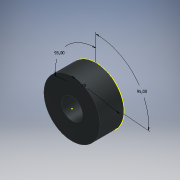
# Autodesk Inventor part: greggio tranciato
Saved by Autodesk Inventor 2018 (Build 220112000, 112)
## iProperties
Created: 2018-08-09
Part Number: greggio tranciato
Material: Ferro, Ghisa grigia ASTM A48 Grado 20
Document SubType Name: Modeling
Designer: carlo
Density: 7.3953 g/cm^3
Appearance: Grigio ferro
Author: carlo
Autodesk Inventor part; units mm, degrees
ref_plane "YZ Plane" through (0, 0, 0) normal (1, 0, 0) x (0, 1, 0)
ref_plane "XZ Plane" through (0, 0, 0) normal (0, 1, 0) x (-1, 0, 0)
ref_plane "XY Plane" through (0, 0, 0) normal (0, 0, 1) x (1, 0, 0)
sketch "Schizzo1" plane through (0, 0, 0) normal (0, 1, 0) x (-1, 0, 0)
  circle A0 centre (0, 0) radius 15
  circle A1 centre (0, 0) radius 40
  dimension "d0" = 30
  dimension "d1" = 80
  constraints: 2 centre point, 2 coincident
  measures "d0" diameter of A0
  measures "d1" diameter of A1
extrude "Estrusione1" add sketch "Schizzo1" against normal blind 34
sketch "Schizzo2" plane through (0, -34, 0) normal (0, -1, 0) x (1, 0, 0)
  point P0 (0, 0)
sketch "Schizzo3" plane through (0, 0, 0) normal (0, 1, 0) x (1, 0, 0)
  circle A0 centre (0, 0) radius 35
  circle A1 centre (0, 0) radius 40 projected
  line L0 (0, -40) -> (0, 0)
  line L1 (0, 0) -> (-39.8478, 3.4862)
  line L2 (0, 0) -> (39.8478, 3.4862)
  point P0 (34.8668, 3.0505)
  point P1 (-34.8668, 3.0505)
  point P2 (0, -35)
  dimension "d4" = 70
  dimension "d5" = 95
  dimension "d6" = 95
  constraints: 6 end point, 6 point on circle, 3 point on line, 1 centre point, 1 coincident, 1 vertical
  measures "d4" diameter of A0
  measures "d5" angle of L1 L0
  measures "d6" angle of L2 L0
